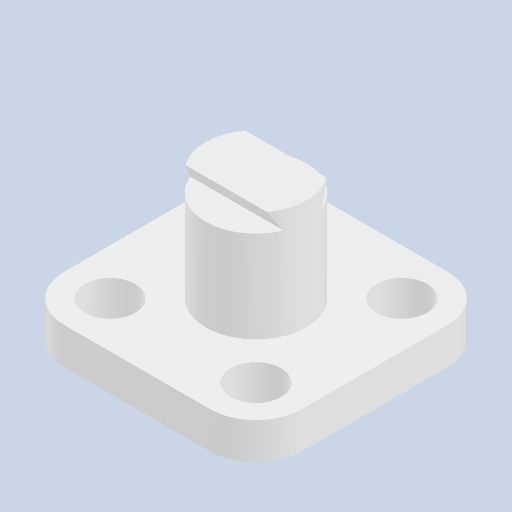
# Autodesk Inventor part: arbore
Saved by Autodesk Inventor 2024 (Build 280153000, 153)
## iProperties
Created: 2023-12-13
Part Number: arbore
Material: Polystyrene
Document SubType Name: Modeling
Designer: mirun
Density: 1.021 g/cm^3
Appearance: Smooth - White
Author: mirun
Autodesk Inventor part; units mm, degrees
ref_plane "YZ Plane" through (0, 0, 0) normal (1, 0, 0) x (0, 1, 0)
ref_plane "XZ Plane" through (0, 0, 0) normal (0, 1, 0) x (-1, 0, 0)
ref_plane "XY Plane" through (0, 0, 0) normal (0, 0, 1) x (1, 0, 0)
sketch "Sketch1" plane through (0, 0, 0) normal (0, 1, 0) x (-1, 0, 0)
  line L0 (7.955, -7.955) -> (-7.955, -7.955)
  line L1 (-7.955, -7.955) -> (-7.955, 7.955)
  line L2 (-7.955, 7.955) -> (7.955, 7.955)
  line L3 (7.955, 7.955) -> (7.955, -7.955)
  circle A0 centre (7.955, -7.955) radius 5
  circle A1 centre (7.955, -7.955) radius 2.75
  line L4 (0, 0) -> (4.4409, 0)
  line L5 (0, 0) -> (0, 4.5835)
  circle A2 centre (7.955, 7.955) radius 5
  circle A3 centre (7.955, 7.955) radius 2.75
  circle A4 centre (-7.955, -7.955) radius 5
  circle A5 centre (-7.955, -7.955) radius 2.75
  circle A6 centre (-7.955, 7.955) radius 2.75
  circle A7 centre (-7.955, 7.955) radius 5
  line L6 (12.955, 7.955) -> (12.955, -7.955)
  line L7 (7.955, -12.955) -> (-7.955, -12.955)
  line L8 (7.955, 12.955) -> (-7.955, 12.955)
  line L9 (-12.955, 7.955) -> (-12.955, -7.955)
  dimension "d0" = 11.25
  dimension "d1" = 10
  dimension "d2" = 5.5
  constraints: 20 end point, 8 centre point, 8 point on circle, 6 coincident, 6 symmetric about line, 6 tangent, 2 horizontal, 2 vertical, 1 parallel, 15 other
  measures "d0" distance of point (0, 0) L0.start
  measures "d1" diameter of A0
  measures "d2" diameter of A1
extrude "Extrusion1" add sketch "Sketch1" along normal blind 4 contours A4 L1 A5 L0 | A4 L1 A7 L2 A2 L3 A0 L0 | L0 A0 L7 A4 | L0 A5 L1 A4 | A0 L3 A1 L0 | L0 A1 L3 A0 | A4 L9 A7 L1 | L3 A2 L6 A0 | A7 L2 A6 L1 | L1 A6 L2 A7 | A2 L2 A3 L3 | L3 A3 L2 A2 | A7 L8 A2 L2
sketch "Sketch3" plane through (0, 4, 0) normal (0, 1, 0) x (1, 0, 0)
  circle A0 centre (0, 0) radius 5.5
  dimension "d26" = 11
  constraints: 1 centre point, 1 coincident
  measures "d26" diameter of A0
extrude "Extrusion4" add sketch "Sketch3" along normal blind 10
sketch "Sketch4" plane through (0, 0, 0) normal (1, 0, 0) x (0, 1, 0)
  line L0 (16, 3.25) -> (16, 0)
  line L1 (16, -3.25) -> (13.638, -1.8863)
  line L2 (16, 3.25) -> (13.9917, 2.0905)
  line L3 (0, 0) -> (20.7938, 0)
  line L4 (16, 0) -> (16, -3.25)
  line L5 (14, -5.5) -> (14, 5.5) construction
  line L6 (13.9917, 2.0905) -> (14, -2.0953)
  dimension "d29" = 60
  dimension "d30" = 60
  dimension "d31" = 2
  dimension "d32" = 6.5
  constraints: 12 end point, 3 point on line, 2 vertical, 1 collinear, 1 horizontal
  measures "d29" angle of L2 L0
  measures "d30" angle of L1 L0
  measures "d31" distance between parallel lines of L5 L0
  measures "d32" distance of L1.start L0.start
extrude "Extrusion5" add sketch "Sketch4" along normal up to surface round surface about axis through (0, 4, 0) along (0, 1, 0) radius 5.5 far side no
extrude "Extrusion6" add sketch "Sketch4" against normal up to surface round surface about axis through (0, 4, 0) along (0, 1, 0) radius 5.5 far side no
body "Solid1"
